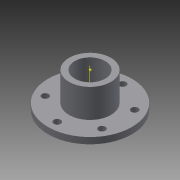
# Autodesk Inventor part: .875 Bearing Hub
Saved by Autodesk Inventor 2014 (Build 180170000, 170)
## iProperties
Created: 2015-01-23
Part Number: .875 Bearing Hub
Material: Generic
Document SubType Name: Modeling
Designer: chappelled
Density: 1 g/cm^3
Appearance: Default
Author: chappelled
Autodesk Inventor part; units mm, degrees
sketch "Sketch1" plane through (0, 0, 0) normal (0, 1, 0) x (-1, 0, 0)
  circle A0 centre (0, 0) radius 30.48
  dimension "d0" = 60.96
  constraints: 1 centre point, 1 coincident
  measures "d0" diameter of A0
extrude "Extrusion1" add sketch "Sketch1" along normal blind 25.4
sketch "Sketch2" plane through (0, 25.4, 0) normal (0, 1, 0) x (1, 0, 0)
  circle A0 centre (0, 0) radius 30.48 projected
  circle A1 centre (0, 0) radius 15.24
  dimension "d3" = 30.48
  constraints: 1 centre point, 1 coincident
  measures "d3" diameter of A1
extrude "Extrusion2" cut sketch "Sketch2" against normal blind 20.828
hole "Hole1" at (0, 25.4, 0) direction (0, -1, 0) diameter 22.225 end through all
ref_plane "Work Plane1" through (0, 0, 23.8252) normal (0, 0, 1) x (1, 0, 0)
hole "Hole2" at (0, 0, 23.8252) direction (0, 1, 0) diameter 5.08 end through all
pattern_circular "Circular Pattern1" count 6 over 360 about axis through (0, 25.4, 0) along (0, -1, 0) of "Hole2"
body "Solid1"
